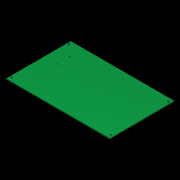
# Autodesk Inventor part: Leiterplatte
Saved by Autodesk Inventor 2011 SP1 (Build 150282100, 282)
## iProperties
Created: 2006-08-30
Part Number: Leiterplatte
Material: Polyaryletherketone Resin
Document SubType Name: Modeling
Designer: becht
Density: 1 g/cm^3
MajorVersion: 11
MinorVersion: 1
Author: becht
Autodesk Inventor part; units mm, degrees
ref_plane "YZ Plane" through (0, 0, 0) normal (1, 0, 0) x (0, 1, 0)
ref_plane "XZ Plane" through (0, 0, 0) normal (0, 1, 0) x (-1, 0, 0)
ref_plane "XY Plane" through (0, 0, 0) normal (0, 0, 1) x (1, 0, 0)
sketch "Skizze1" plane through (0, 0, 0) normal (0, 0, 1) x (1, 0, 0)
  line L0 (0, -93.2598) -> (160, -93.2598)
  line L1 (160, -93.2598) -> (160, 6.7402)
  line L2 (160, 6.7402) -> (0, 6.7402)
  line L3 (0, 6.7402) -> (0, -93.2598)
  circle A0 centre (5.4, -3.8898) radius 0.4
  point P0 (2.5, 1.1902)
  point P1 (156.5, 1.1902)
  point P2 (2.5, -87.7098)
  point P3 (156.5, -87.7598)
  point P4 (19.5566, -14.9779)
  dimension "d0" = 160
  dimension "d1" = 100
  dimension "d146" = 0.8
  dimension "d147" = 5.4
  dimension "d148" = 10.63
  dimension "d162" = 5.55
  dimension "d163" = 2.5
  dimension "d164" = 154
  dimension "d165" = 88.9
  dimension "d194" = 5.55
  constraints: 8 end point, 2 parallel, 1 centre point, 1 horizontal, 1 perpendicular
  measures "d0" distance of L1.end L2.end
  measures "d1" distance of L2.end L0.start
  measures "d146" diameter of A0
  measures "d147" distance from line of A0.centre L3
  measures "d148" distance from line of A0.centre L2
  measures "d162" distance from line of L2 point (2.5, 1.19)
  measures "d163" distance from line of L3 point (2.5, 1.19)
  measures "d164" distance of point (2.5, 1.19) point (156.5, 1.19)
  measures "d165" distance of point (2.5, 1.19) point (2.5, -87.71)
  measures "d194" distance from line of L0 point (2.5, -87.71)
extrude "Extrusion1" add sketch "Skizze1" along normal blind 1.6 contours L3 L2 L1 L0 | A0
sketch "Skizze2" plane through (0, 0, 1.6) normal (0, 0, 1) x (1, 0, 0)
  line L0 (0, -93.2598) -> (0, 6.7402) projected
  line L1 (4.4, -2.8898) -> (6.4, -2.8898)
  line L2 (6.4, -2.8898) -> (6.4, -4.8898)
  line L3 (6.4, -4.8898) -> (4.4, -4.8898)
  line L4 (4.4, -4.8898) -> (4.4, -2.8898)
  line L5 (0, 6.7402) -> (160, 6.7402) projected
  dimension "d4" = 2
  dimension "d5" = 2
  dimension "d7" = 4.4
  dimension "d145" = 9.63
  constraints: 8 end point, 2 parallel, 1 horizontal, 1 perpendicular
  measures "d4" distance of L1.start L1.end
  measures "d5" distance of L3.end L1.start
  measures "d7" distance between parallel lines of L0 L4
  measures "d145" distance between parallel lines of L5 L1
hole "Bohrung12" at (2.5, 1.1902, 0) at (156.5, 1.1902, 0) at (2.5, -87.7098, 0) at (156.5, -87.7598, 0) direction (0, 0, 1) diameter 3 end through all
sketch "Skizze7" plane through (0, 0, 0) normal (0, 0, -1) x (-1, 0, 0)
  circle A0 centre (-19.677, -14.9883) radius 1.0356
  point P0 (0, 0)
  constraints: 1 centre point, 1 coincident
hole "Hole14" at (19.677, -14.9883, 0) direction (0, 0, 1) diameter 2 depth 4 tip angle 118
sketch "Skizze8" plane through (0, 0, 1.6) normal (0, 0, 1) x (1, 0, 0)
  point P0 (0, 0)
  point P1 (19.4698, -35.0394)
hole "Hole15" at (19.4698, -35.0394, 1.6) direction (0, 0, -1) diameter 2 depth 4 tip angle 118
